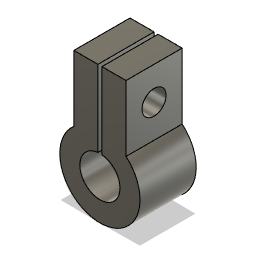
_Shaft Clamp.192d11ff-f064-4aea-b497-f171f266d952 (Autodesk Fusion 360 design; units mm, degrees)
Autodesk Fusion 360 part; units mm, degrees
sketch "Sketch1" plane through (0, 0, 0) normal (0, 0, 1) x (1, 0, 0)
  circle A0 centre (0, 0) radius 5
  circle A1 centre (0, 0) radius 2.5
  line L0 (-3.25, 3.7997) -> (-3.25, 12)
  line L1 (-3.25, 12) -> (-0.25, 12)
  line L2 (0.25, 12) -> (3.25, 12)
  line L3 (3.25, 12) -> (3.25, 3.7997)
  line L4 (-0.25, 12) -> (-0.25, 2.4875)
  line L5 (0.25, 12) -> (0.25, 2.4875)
  line L6 (0.25, 7.2437) -> (-0.25, 7.2437) construction
  line L7 (0, 7.2437) -> (0, 0) construction
  dimension "d1" = 10
  dimension "d2" = 5
  dimension "d3" = 3
  dimension "d4" = 3
  dimension "d5" = 0.5
  dimension "d6" = 12
  constraint coincident A0.centre A1.centre
  constraint concentric A0 A1
  constraint coincident A0 L0.start
  constraint vertical L0
  constraint perpendicular L0 L1
  constraint coincident A0 L3.end
  constraint perpendicular L2 L3
  constraint coincident A1 L4.end
  constraint perpendicular L1 L4
  constraint coincident A1 L5.end
  constraint perpendicular L1 L5
  constraint horizontal L2
  constraint midpoint L5 L6.start
  constraint coincident L4 L6.end
  constraint perpendicular L4 L6
  constraint midpoint L6 L7.start
  constraint vertical L7
  constraint collinear L1 L2
  measures "d1" diameter of A0
  measures "d2" diameter of A1
  measures "d3" distance of L0 L4
  measures "d4" horizontal distance of L2.start L2.end
  measures "d5" distance of L4 L5
  measures "d6" distance of A0.centre L1
extrude "Extrude1" add sketch "Sketch1" along normal blind 7 contours A0 A1 L4 L5 | A0 L2 L3 L5 | A0 L0 L1 L4 picked at (-2.9647, 2.9128)
sketch "Sketch2" plane through (-3.25, 0, 0) normal (-1, 0, 0) x (0, 0, 1)
  line L0 (0, 12) -> (0, 3.7997)
  line L1 (0, 3.7997) -> (7, 3.7997)
  line L2 (7, 3.7997) -> (7, 12)
  line L3 (7, 12) -> (0, 12)
  line L4 (0, 12) -> (7, 3.7997) construction
  circle A0 centre (3.5, 7.8998) radius 1.5
  dimension "d9" = 3
  constraint coincident L0.start L3.end
  constraint coincident L1.end L2.start
  constraint midpoint L4 A0.centre
  measures "d9" diameter of A0
extrude "Extrude2" cut sketch "Sketch2" against normal blind 6.5 contours A0
